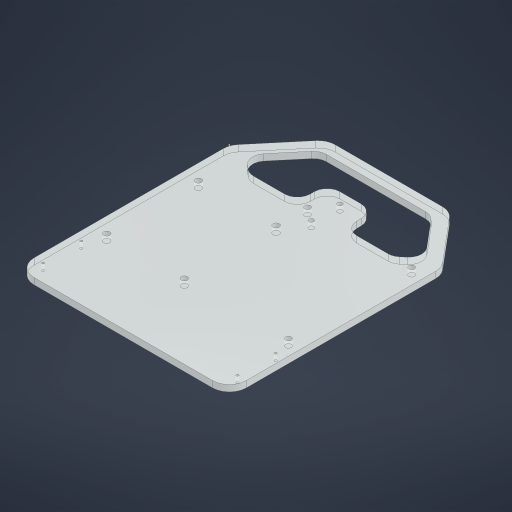
# Autodesk Inventor part: ROBOT CHASSIS PLATE
Saved by Autodesk Inventor 2023 (Build 270158000, 158)
## iProperties
Created: 2023-03-03
Part Number: ROBOT CHASSIS PLATE
Material: Generic
Document SubType Name: Modeling
Designer: Phoenix
Density: 1 g/cm^3
Appearance: Clear
Author: Phoenix
Autodesk Inventor part; units mm, degrees
ref_plane "YZ Plane" through (0, 0, 0) normal (1, 0, 0) x (0, 1, 0)
ref_plane "XZ Plane" through (0, 0, 0) normal (0, 1, 0) x (-1, 0, 0)
ref_plane "XY Plane" through (0, 0, 0) normal (0, 0, 1) x (1, 0, 0)
sketch "Sketch1" plane through (0, 0, 0) normal (0, 1, 0) x (-1, 0, 0)
  line L0 (0, 0) -> (-100, 0) construction
  line L1 (-100, 0) -> (-100, 100)
  line L2 (-100, 100) -> (0, 100)
  line L3 (0, 100) -> (0, 0)
  circle A0 centre (-4.25, 92) radius 0.575
  circle A1 centre (-4.25, 74) radius 0.575
  line L4 (-50, 100) -> (-50, 0) construction
  line L5 (-7.212, 21.82) -> (-7.212, 65) construction
  line L6 (-7.212, 65) -> (-43.788, 65) construction
  line L7 (-7.212, 21.82) -> (-43.788, 21.82) construction
  circle A2 centre (-7.212, 65) radius 1.5
  circle A3 centre (-43.788, 65) radius 1.5
  circle A4 centre (-7.212, 21.82) radius 1.5
  circle A5 centre (-43.788, 21.82) radius 1.5
  line L8 (-43.788, 7) -> (-92.788, 7) construction
  line L9 (-92.788, 7) -> (-92.788, 65) construction
  line L10 (-92.788, 65) -> (-43.788, 65) construction
  line L11 (-43.788, 65) -> (-43.788, 7) construction
  circle A6 centre (-43.788, 7) radius 1.375
  circle A7 centre (-92.788, 7) radius 1.375
  circle A8 centre (-92.788, 65) radius 1.375
  circle A9 centre (-43.788, 65) radius 1.375
  line L12 (-7.212, 43.41) -> (0, 43.41) construction
  line L13 (-92.788, 36) -> (-100, 36) construction
  line L14 (0, 0) -> (-100, 0) construction
  circle A10 centre (-95.75, 74) radius 0.575
  circle A11 centre (-95.75, 92) radius 0.575
  line L15 (-39, 7) -> (-61, 7)
  line L16 (-61, 7) -> (-61, -7)
  line L17 (-61, -7) -> (-39, -7)
  line L18 (-39, -7) -> (-39, 7)
  line L19 (-39, 7) -> (-61, -7) construction
  line L20 (-61, 7) -> (-39, -7) construction
  line L21 (-50, 0) -> (-50, -25) construction
  line L22 (-50, -25) -> (-20.9775, -25)
  line L23 (-20.9775, -25) -> (0, 0)
  line L24 (-7.8324, 0) -> (-23.7753, -19)
  line L25 (-23.7753, -19) -> (-50, -19)
  line L26 (-39, 7) -> (-16.1201, 7)
  line L27 (-16.1201, 7) -> (-7.8324, 0)
  line L28 (-50, -25) -> (-79.0225, -25)
  line L29 (-79.0225, -25) -> (-100, 0)
  line L30 (-92.1676, 0) -> (-76.2247, -19)
  line L31 (-76.2247, -19) -> (-50, -19)
  line L32 (-61, 7) -> (-83.8799, 7)
  line L33 (-83.8799, 7) -> (-92.1676, 0)
  line L34 (-30, 100) -> (-70, 100)
  line L35 (-50, -2) -> (-50, 11.462) construction
  circle A12 centre (-50, -2) radius 1.15
  circle A13 centre (-50, 11.462) radius 1.15
  point P0 (-50, 80)
  point P1 (-50, 4.731)
  dimension "d0" = 100
  dimension "d1" = 100
  dimension "d2" = 8
  dimension "d3" = 4.25
  dimension "d4" = 1.15
  dimension "d5" = 18
  dimension "d6" = 43.18
  dimension "d7" = 36.576
  dimension "d8" = 3
  dimension "d9" = 49
  dimension "d10" = 58
  dimension "d15" = 2.75
  dimension "d33" = 22
  dimension "d34" = 25
  dimension "d36" = 130
  dimension "d37" = 6
  dimension "d38" = 6
  dimension "d39" = 14
  dimension "d44" = 2.3
  dimension "d45" = 13.462
  dimension "d46" = 5
  constraints: 72 end point, 14 centre point, 11 coincident, 9 parallel, 8 equal radius, 8 horizontal, 8 point on line, 7 midpoint, 7 perpendicular, 7 symmetric about line, 3 vertical, 2 other
  measures "d0" distance of L1.end L2.end
  measures "d1" distance of L0.end L1.end
  measures "d2" distance from line of L2 point (-4.25, 92)
  measures "d3" distance from line of L3 point (-4.25, 92)
  measures "d4" diameter of A0
  measures "d5" distance of A0.centre A1.centre
  measures "d6" distance of L5.end L5.start
  measures "d7" distance of L5.end L6.end
  measures "d8" diameter of A2
  measures "d9" distance of L6.end L9.end
  measures "d10" distance of L8.end L9.end
  measures "d15" diameter of A8
  measures "d33" distance of L17.end L16.end
  measures "d34" distance of L4.end L21.end
  measures "d36" angle of L0 L23
  measures "d37" distance between parallel lines of L23 L24
  measures "d38" distance between parallel lines of L22 L25
  measures "d39" distance of L17.end L15.start
  measures "d44" diameter of A12
  measures "d45" distance of L35.end L35.start
  measures "d46" distance from line of L17 A12.centre
extrude "Extrusion1" add sketch "Sketch1" along normal blind 3 contours L1 L2 L3 L23 L22 L28 L29 | L15 L18 L17 L16 A6
fillet "Fillet1" radius 6 10 edges at (61, 1.5, 7) (39, 1.5, 7) (39, 1.5, -7) (61, 1.5, -7) (7.8324, 1.5, 0) (92.1676, 1.5, 0) (83.8799, 1.5, 7) (16.1201, 1.5, 7) (23.7753, 1.5, -19) (76.2247, 1.5, -19)
fillet "Fillet1" radius 8 6 edges at (20.9775, 1.5, -25) (0, 1.5, 0) (79.0225, 1.5, -25) (100, 1.5, 0) (100, 1.5, 100) (0, 1.5, 100)
sketch "Sketch2" plane through (0, 3, 0) normal (0, 1, 0) x (1, 0, 0)
  point P0 (0, 0)
body "Solid1"
